Autodesk Fusion 360 part; units mm, degrees
note: some values were not read from the file. Chosen so that the rebuilt part matches the saved one: which bodies a step acts on; which face or edge a step refers to. Set by a fixed rule: which sketch regions a step uses.
(part 3 of 4)
sketch "Profile (3)" plane through (0, 0, 21) normal (0, 0, 1) x (-1, 0, 0) in component "Top Plate"
  circle A0 centre (172.0478, -239.295) radius 1.5
  circle A1 centre (168.5847, -232.6424) radius 5
  circle A2 centre (165.1216, -225.9898) radius 1.5
  circle A3 centre (67, -37.5) radius 1.5
  circle A4 centre (78.7284, -60.0301) radius 1.5
  line L0 (167.0843, -250.3342) -> (183.9375, -241.5609)
  line L1 (183.9375, -241.5609) -> (73.1179, -28.6783)
  line L2 (73.1179, -28.6783) -> (56.2647, -37.4516)
  line L3 (56.2647, -37.4516) -> (167.0843, -250.3342)
  line L4 (156, -22.3832) -> (156, 22.3832)
  arc A5 (155.0534, -25.3107) -> (156, -22.3832) centre (151, -22.3832) ccw
  line L5 (150.3466, -31.8278) -> (155.0534, -25.3107)
  arc A6 (148.1584, -33.5394) -> (150.3466, -31.8278) centre (146.2932, -28.9003) ccw
  line L6 (102.5293, -51.8851) -> (148.1584, -33.5394)
  arc A7 (102.5293, -51.8851) -> (100.1362, -53.9037) centre (104.3945, -56.5242) ccw
  line L7 (94.075, -63.7531) -> (100.1362, -53.9037)
  arc A8 (91.0078, -65.9886) -> (94.075, -63.7531) centre (89.8167, -61.1326) ccw
  line L8 (68.4899, -71.5119) -> (91.0078, -65.9886)
  arc A9 (64.7398, -70.9514) -> (68.4899, -71.5119) centre (67.2988, -66.6559) ccw
  line L9 (43.9667, -58.5759) -> (64.7398, -70.9514)
  arc A10 (43.9667, -58.5759) -> (41.8797, -57.8938) centre (41.4077, -62.8714) ccw
  line L10 (-13.2682, -52.6642) -> (41.8797, -57.8938)
  arc A11 (-13.2682, -52.6642) -> (-16.4597, -53.4461) centre (-13.7403, -57.6419) ccw
  line L11 (-40.2244, -68.8491) -> (-16.4597, -53.4461)
  arc A12 (-44.0623, -69.5267) -> (-40.2244, -68.8491) centre (-42.9439, -64.6534) ccw
  line L12 (-71.0992, -63.3215) -> (-44.0623, -69.5267)
  arc A13 (-73.5163, -61.9837) -> (-71.0992, -63.3215) centre (-69.9807, -58.4482) ccw
  line L13 (-87.8503, -47.6497) -> (-73.5163, -61.9837)
  arc A14 (-87.8503, -47.6497) -> (-90.606, -46.2464) centre (-91.3858, -51.1852) ccw
  line L14 (-143.7908, -37.8488) -> (-90.606, -46.2464)
  arc A15 (-147.2125, -35.6206) -> (-143.7908, -37.8488) centre (-143.011, -32.91) ccw
  line L15 (-155.2015, -23.2377) -> (-147.2125, -35.6206)
  arc A16 (-156, -20.5271) -> (-155.2015, -23.2377) centre (-151, -20.5271) ccw
  line L16 (-156, 20.5271) -> (-156, -20.5271)
  arc A17 (-155.2015, 23.2377) -> (-156, 20.5271) centre (-151, 20.5271) ccw
  line L17 (-147.2125, 35.6206) -> (-155.2015, 23.2377)
  arc A18 (-143.7908, 37.8488) -> (-147.2125, 35.6206) centre (-143.011, 32.91) ccw
  line L18 (-90.606, 46.2464) -> (-143.7908, 37.8488)
  arc A19 (-90.606, 46.2464) -> (-87.8503, 47.6497) centre (-91.3858, 51.1852) ccw
  circle A20 centre (-90.7, 41.475) radius 1.5
  line L19 (-73.5163, 61.9837) -> (-87.8503, 47.6497)
  arc A21 (-71.0992, 63.3215) -> (-73.5163, 61.9837) centre (-69.9807, 58.4482) ccw
  line L20 (-44.0623, 69.5267) -> (-71.0992, 63.3215)
  circle A22 centre (-56.2284, 60.0301) radius 1.5
  circle A23 centre (-44.5, 37.5) radius 1.5
  arc A24 (-40.2244, 68.8491) -> (-44.0623, 69.5267) centre (-42.9439, 64.6534) ccw
  line L21 (-16.4597, 53.4461) -> (-40.2244, 68.8491)
  arc A25 (-16.4597, 53.4461) -> (-13.2682, 52.6642) centre (-13.7403, 57.6419) ccw
  line L22 (41.8797, 57.8938) -> (-13.2682, 52.6642)
  arc A26 (41.8797, 57.8938) -> (43.9667, 58.5759) centre (41.4077, 62.8714) ccw
  line L23 (64.7398, 70.9514) -> (43.9667, 58.5759)
  arc A27 (68.4899, 71.5119) -> (64.7398, 70.9514) centre (67.2988, 66.6559) ccw
  line L24 (91.0078, 65.9886) -> (68.4899, 71.5119)
  arc A28 (94.075, 63.7531) -> (91.0078, 65.9886) centre (89.8167, 61.1326) ccw
  line L25 (100.1362, 53.9037) -> (94.075, 63.7531)
  circle A29 centre (78.7284, 60.0301) radius 1.5
  circle A30 centre (67, 37.5) radius 1.5
  arc A31 (100.1362, 53.9037) -> (102.5293, 51.8851) centre (104.3945, 56.5242) ccw
  line L26 (148.1584, 33.5394) -> (102.5293, 51.8851)
  circle A32 centre (101.7, 47.55) radius 1.5
  arc A33 (150.3466, 31.8278) -> (148.1584, 33.5394) centre (146.2932, 28.9003) ccw
  line L27 (155.0534, 25.3107) -> (150.3466, 31.8278)
  arc A34 (156, 22.3832) -> (155.0534, 25.3107) centre (151, 22.3832) ccw
  circle A35 centre (151.35, 22.65) radius 1.5
  circle A36 centre (151.35, -22.65) radius 1.5
  circle A37 centre (101.7, -47.55) radius 1.5
  circle A38 centre (78.7284, -60.0301) radius 1.5
  circle A39 centre (67, -37.5) radius 1.5
  circle A40 centre (-44.5, -37.5) radius 1.5
  circle A41 centre (-56.2284, -60.0301) radius 1.5
  circle A42 centre (-90.7, -41.475) radius 1.5
  circle A43 centre (-151.5, -21.3) radius 1.5
  circle A44 centre (-151.5, 21.3) radius 1.5
  line L28 (155.6622, 0) -> (-156.3378, 0) construction
  line L29 (52, 0) -> (52, -20.8972)
  line L30 (49.8679, -24.9929) -> (34.3684, -35.8458)
  line L31 (31.5005, -36.75) -> (-11.9635, -36.75)
  line L32 (-13.7553, -36.4179) -> (-40.2918, -26.2315)
  line L33 (-43.5, -21.5636) -> (-43.5, 0)
  arc A45 (-43.5, -21.5636) -> (-40.2918, -26.2315) centre (-38.5, -21.5636) ccw
  arc A46 (-13.7553, -36.4179) -> (-11.9635, -36.75) centre (-11.9635, -31.75) ccw
  arc A47 (31.5005, -36.75) -> (34.3684, -35.8458) centre (31.5005, -31.75) ccw
  arc A48 (49.8679, -24.9929) -> (52, -20.8972) centre (47, -20.8972) ccw
  line L34 (52, 0) -> (52, 20.8972)
  arc A49 (52, 20.8972) -> (49.8679, 24.9929) centre (47, 20.8972) ccw
  line L35 (49.8679, 24.9929) -> (34.3684, 35.8458)
  arc A50 (34.3684, 35.8458) -> (31.5005, 36.75) centre (31.5005, 31.75) ccw
  line L36 (31.5005, 36.75) -> (-11.9635, 36.75)
  arc A51 (-11.9635, 36.75) -> (-13.7553, 36.4179) centre (-11.9635, 31.75) ccw
  line L37 (-13.7553, 36.4179) -> (-40.2918, 26.2315)
  arc A52 (-40.2918, 26.2315) -> (-43.5, 21.5636) centre (-38.5, 21.5636) ccw
  line L38 (-43.5, 21.5636) -> (-43.5, 0)
  circle A53 centre (151.35, 22.65) radius 3.2
  circle A54 centre (151.35, 22.65) radius 1.7
  circle A55 centre (151.35, -22.65) radius 3.2
  circle A56 centre (151.35, -22.65) radius 1.7
  circle A57 centre (101.7, 47.55) radius 3.2
  circle A58 centre (101.7, 47.55) radius 1.7
  circle A59 centre (-90.7, 41.475) radius 3.2
  circle A60 centre (-90.7, 41.475) radius 1.7
  circle A61 centre (-151.5, 21.3) radius 3.2
  circle A62 centre (-151.5, 21.3) radius 1.7
  circle A63 centre (-151.5, -21.3) radius 3.2
  circle A64 centre (-151.5, -21.3) radius 1.7
  circle A65 centre (-90.7, -41.475) radius 3.2
  circle A66 centre (-90.7, -41.475) radius 1.7
  circle A67 centre (101.7, -47.55) radius 3.2
  circle A68 centre (101.7, -47.55) radius 1.7
  point P0 (52, -23.5)
  point P1 (-43.5, -25)
  dimension "d210" = 95.5
  dimension "d211" = 43.5
  dimension "d212" = 36.75
  dimension "d213" = 25
  dimension "d214" = 23.5
  dimension "d215" = 145
  dimension "d216" = 159
  dimension "d217" = 5
  dimension "d218" = 5
  dimension "d219" = 5
  dimension "d220" = 5
  dimension "d339" = 6.4
  dimension "d340" = 3.4
  dimension "d341" = 6.4
  dimension "d342" = 3.4
  dimension "d343" = 6.4
  dimension "d344" = 3.4
  dimension "d345" = 6.4
  dimension "d346" = 3.4
  dimension "d347" = 6.4
  dimension "d348" = 3.4
  dimension "d349" = 6.4
  dimension "d350" = 3.4
  dimension "d351" = 6.4
  dimension "d352" = 3.4
  dimension "d353" = 6.4
  dimension "d354" = 3.4
  constraint coincident origin L28
  constraint coincident L28 L29.start
  constraint coincident L28 L33.end
  constraint vertical L29
  constraint vertical L33
  constraint horizontal L31
  constraint coincident P1 L32
  constraint coincident P1 L33
  constraint tangent L32 A45
  constraint tangent L33 A45
  constraint tangent L31 A46
  constraint tangent L32 A46
  constraint tangent L30 A47
  constraint tangent L31 A47
  constraint coincident P0 L29
  constraint coincident P0 L30
  constraint tangent L29 A48
  constraint tangent L30 A48
  constraint symmetric L28 L29.start L34.start
  constraint symmetric L28 L33.end L38.end
  constraint symmetric L28 L32.end L37.end
  constraint symmetric L28 L33.start A52.end
  constraint symmetric L28 A45 A52
  constraint symmetric L28 L31.end L36.end
  constraint symmetric L28 L32.start A51.end
  constraint symmetric L28 A46 A51
  constraint symmetric L28 L30.end L35.end
  constraint symmetric L28 L31.start A50.end
  constraint symmetric L28 A47 A50
  constraint symmetric L28 L29.end L34.end
  constraint symmetric L28 L30.start A49.end
  constraint symmetric L28 A48 A49
  constraint concentric A35 A53
  constraint concentric A53 A54
  constraint concentric A36 A55
  constraint concentric A55 A56
  constraint concentric A32 A57
  constraint concentric A57 A58
  constraint concentric A20 A59
  constraint concentric A59 A60
  constraint concentric A44 A61
  constraint concentric A61 A62
  constraint concentric A43 A63
  constraint concentric A63 A64
  constraint concentric A42 A65
  constraint concentric A65 A66
  constraint concentric A37 A67
  constraint concentric A67 A68
  measures "d210" distance of P0 L33
  measures "d211" distance of origin L33
  measures "d212" distance of L28 L31
  measures "d213" distance of P1 L33.end
  measures "d214" distance of L29.start P0
  measures "d215" angle of L30 L31
  measures "d216" angle of L31 L32
  measures "d217" radius of A45
  measures "d218" radius of A46
  measures "d219" radius of A47
  measures "d220" radius of A48
  measures "d339" diameter of A53
  measures "d340" diameter of A54
  measures "d341" diameter of A55
  measures "d342" diameter of A56
  measures "d343" diameter of A57
  measures "d344" diameter of A58
  measures "d345" diameter of A59
  measures "d346" diameter of A60
  measures "d347" diameter of A61
  measures "d348" diameter of A62
  measures "d349" diameter of A63
  measures "d350" diameter of A64
  measures "d351" diameter of A65
  measures "d352" diameter of A66
  measures "d353" diameter of A67
  measures "d354" diameter of A68
extrude "Extrude1''''" add sketch "Profile (3)" along normal blind 2 separate body contours L1 L2 L3 L4 A5 L5 A6 L6 A7 L7 A8 L8 A9 L9 A10 L10 A11 L11 A12 L12 A13 L13 A14 L14 A15 L15 A16 L16 A17 L17 A18 L18 A19 L19 A21 L20 A24 L21 A25 L22 A26 L23 A27 L24 A28 L25 A31 L26 A33 L27 A34 | L1 L2 L3 A8 L8 | A53 | A54 | A55 | A56 | A57 | A58 | A59 | A60 | A61 | A62 | A63 | A64 | A65 | A66 | A67 | A68 makes body 39 in component "Top Plate"
ref_plane "WorkPlane1" through (0, 0, 33) normal (0, 0, 1) x (-1, 0, 0)
ref_plane "WorkPlane2" through (0, 0, 50) normal (0, 0, 1) x (-1, 0, 0)
sketch "Profile (4)" plane through (0, 0, 33) normal (0, 0, 1) x (1, 0, 0) in component "Pixhawk Plate"
  line L0 (-96.5, 0) -> (76.5, 0) construction
  line L1 (-96.5, 0) -> (-96.5, 20.5093)
  line L2 (-95.8379, 21.9959) -> (-82.5, 34)
  line L3 (-82.5, 34) -> (-79.0886, 42.1448)
  line L4 (-77.0182, 43.9038) -> (-62.67, 47.3296)
  line L5 (-58.958, 46.7668) -> (-50.5, 41.75)
  line L6 (-50.5, 41.75) -> (17.5, 36.3)
  line L7 (17.5, 36.3) -> (35.25, 47.75)
  line L8 (35.25, 47.75) -> (38.75, 47.75)
  line L9 (38.75, 47.75) -> (51.4852, 44.6807)
  line L10 (52.952, 43.2406) -> (55.75, 32.5)
  line L11 (55.75, 32.5) -> (76.5, 21)
  line L12 (76.5, 21) -> (76.5, 0)
  arc A0 (-95.8379, 21.9959) -> (-96.5, 20.5093) centre (-94.5, 20.5093) ccw
  arc A1 (-77.0182, 43.9038) -> (-79.0886, 42.1448) centre (-76.3215, 40.9858) ccw
  arc A2 (-58.958, 46.7668) -> (-62.67, 47.3296) centre (-61.5088, 42.4663) ccw
  arc A3 (52.952, 43.2406) -> (51.4852, 44.6807) centre (51.0166, 42.7364) ccw
  circle A4 centre (-67, 37.5) radius 1.5
  circle A5 centre (44.5, 37.5) radius 1.5
  circle A6 centre (44.5, -37.5) radius 1.5
  circle A7 centre (-67, -37.5) radius 1.5
  line L13 (-80.8, 26.9) -> (-67.05, 26.9)
  line L14 (-67.05, 22.65) -> (-80.8, 22.65)
  line L15 (-25.375, 30.5) -> (-7.875, 30.5)
  line L16 (-7.875, 26.25) -> (-25.375, 26.25)
  line L17 (4.975, 30.5) -> (17.375, 30.5)
  line L18 (17.375, 26.25) -> (4.975, 26.25)
  line L19 (43.3, 24.8) -> (59.3, 24.8)
  line L20 (59.3, 20.55) -> (43.3, 20.55)
  line L21 (32.35, 0) -> (32.35, 20.5)
  line L22 (37.1, 20.5) -> (37.1, 0)
  line L23 (-59, 0) -> (-59, 20)
  line L24 (-54.25, 20) -> (-54.25, 0)
  circle A8 centre (-42.25, 34) radius 1.5
  circle A9 centre (28.4, 34) radius 1.5
  circle A10 centre (39.175, 41.335) radius 1.5
  arc A11 (59.3, 20.55) -> (59.3, 24.8) centre (59.3, 22.675) ccw
  arc A12 (43.3, 24.8) -> (43.3, 20.55) centre (43.3, 22.675) ccw
  arc A13 (37.1, 20.5) -> (32.35, 20.5) centre (34.725, 20.5) ccw
  arc A14 (-25.375, 30.5) -> (-25.375, 26.25) centre (-25.375, 28.375) ccw
  arc A15 (-7.875, 26.25) -> (-7.875, 30.5) centre (-7.875, 28.375) ccw
  arc A16 (4.975, 30.5) -> (4.975, 26.25) centre (4.975, 28.375) ccw
  arc A17 (17.375, 26.25) -> (17.375, 30.5) centre (17.375, 28.375) ccw
  arc A18 (-80.8, 26.9) -> (-80.8, 22.65) centre (-80.8, 24.775) ccw
  arc A19 (-67.05, 22.65) -> (-67.05, 26.9) centre (-67.05, 24.775) ccw
  arc A20 (-54.25, 20) -> (-59, 20) centre (-56.625, 20) ccw
  line L25 (-42.25, 34) -> (28.4, 34) construction
  arc A21 (-59, -20) -> (-54.25, -20) centre (-56.625, -20) ccw
  line L26 (-7.875, -26.25) -> (-25.375, -26.25)
  line L27 (-54.25, -20) -> (-54.25, 0)
  line L28 (35.25, -47.75) -> (38.75, -47.75)
  line L29 (-50.5, -41.75) -> (17.5, -36.3)
  arc A22 (59.3, -24.8) -> (59.3, -20.55) centre (59.3, -22.675) ccw
  circle A23 centre (-42.25, -34) radius 1.5
  line L30 (-42.25, -34) -> (28.4, -34) construction
  arc A24 (32.35, -20.5) -> (37.1, -20.5) centre (34.725, -20.5) ccw
  arc A25 (-79.0886, -42.1448) -> (-77.0182, -43.9038) centre (-76.3215, -40.9858) ccw
  arc A26 (4.975, -26.25) -> (4.975, -30.5) centre (4.975, -28.375) ccw
  line L31 (32.35, 0) -> (32.35, -20.5)
  line L32 (-58.958, -46.7668) -> (-50.5, -41.75)
  line L33 (-77.0182, -43.9038) -> (-62.67, -47.3296)
  arc A27 (-67.05, -26.9) -> (-67.05, -22.65) centre (-67.05, -24.775) ccw
  line L34 (-59, 0) -> (-59, -20)
  arc A28 (-25.375, -26.25) -> (-25.375, -30.5) centre (-25.375, -28.375) ccw
  line L35 (-96.5, 0) -> (-96.5, -20.5093)
  arc A29 (-62.67, -47.3296) -> (-58.958, -46.7668) centre (-61.5088, -42.4663) ccw
  line L36 (-25.375, -30.5) -> (-7.875, -30.5)
  arc A30 (-80.8, -22.65) -> (-80.8, -26.9) centre (-80.8, -24.775) ccw
  arc A31 (43.3, -20.55) -> (43.3, -24.8) centre (43.3, -22.675) ccw
  circle A32 centre (44.5, -37.5) radius 1.5
  line L37 (4.975, -30.5) -> (17.375, -30.5)
  arc A33 (17.375, -30.5) -> (17.375, -26.25) centre (17.375, -28.375) ccw
  arc A34 (-7.875, -30.5) -> (-7.875, -26.25) centre (-7.875, -28.375) ccw
  circle A35 centre (28.4, -34) radius 1.5
  line L38 (59.3, -20.55) -> (43.3, -20.55)
  line L39 (37.1, -20.5) -> (37.1, 0)
  line L40 (-67.05, -22.65) -> (-80.8, -22.65)
  circle A36 centre (-67, -37.5) radius 1.5
  arc A37 (-96.5, -20.5093) -> (-95.8379, -21.9959) centre (-94.5, -20.5093) ccw
  line L41 (-80.8, -26.9) -> (-67.05, -26.9)
  line L42 (17.5, -36.3) -> (35.25, -47.75)
  line L43 (-82.5, -34) -> (-79.0886, -42.1448)
  line L44 (76.5, -21) -> (76.5, 0)
  arc A38 (51.4852, -44.6807) -> (52.952, -43.2406) centre (51.0166, -42.7364) ccw
  line L45 (55.75, -32.5) -> (76.5, -21)
  line L46 (52.952, -43.2406) -> (55.75, -32.5)
  line L47 (43.3, -24.8) -> (59.3, -24.8)
  circle A39 centre (39.175, -41.335) radius 1.5
  line L48 (38.75, -47.75) -> (51.4852, -44.6807)
  line L49 (-95.8379, -21.9959) -> (-82.5, -34)
  line L50 (17.375, -26.25) -> (4.975, -26.25)
  circle A40 centre (-67, 37.5) radius 2.75 construction
  line L51 (-67, 40.25) -> (-67, 34.75) construction
  line L52 (-64.25, 37.5) -> (-69.75, 37.5) construction
  line L53 (-64.6184, 38.875) -> (-64.6184, 36.125)
  line L54 (-67, 34.75) -> (-64.6184, 36.125)
  line L55 (-64.6184, 38.875) -> (-67, 40.25)
  line L56 (-69.3816, 38.875) -> (-69.3816, 36.125)
  line L57 (-69.3816, 38.875) -> (-67, 40.25)
  line L58 (-67, 34.75) -> (-69.3816, 36.125)
  circle A41 centre (-67, 37.5) radius 1.25
  line L59 (46.8816, 38.875) -> (44.5, 40.25)
  line L60 (42.1184, 38.875) -> (44.5, 40.25)
  line L61 (44.5, 34.75) -> (42.1184, 36.125)
  line L62 (44.5, 40.25) -> (44.5, 34.75) construction
  line L63 (46.8816, 38.875) -> (46.8816, 36.125)
  circle A42 centre (44.5, 37.5) radius 2.75 construction
  circle A43 centre (44.5, 37.5) radius 1.25
  line L64 (47.25, 37.5) -> (41.75, 37.5) construction
  line L65 (42.1184, 38.875) -> (42.1184, 36.125)
  line L66 (44.5, 34.75) -> (46.8816, 36.125)
  line L67 (-67, -34.75) -> (-67, -40.25) construction
  line L68 (-69.3816, -36.125) -> (-67, -34.75)
  line L69 (-64.25, -37.5) -> (-69.75, -37.5) construction
  circle A44 centre (-67, -37.5) radius 2.75 construction
  line L70 (-69.3816, -36.125) -> (-69.3816, -38.875)
  line L71 (-64.6184, -36.125) -> (-67, -34.75)
  line L72 (-67, -40.25) -> (-64.6184, -38.875)
  line L73 (-67, -40.25) -> (-69.3816, -38.875)
  circle A45 centre (-67, -37.5) radius 1.25
  line L74 (-64.6184, -36.125) -> (-64.6184, -38.875)
  line L75 (44.5, -34.75) -> (44.5, -40.25) construction
  line L76 (42.1184, -36.125) -> (44.5, -34.75)
  line L77 (46.8816, -36.125) -> (44.5, -34.75)
  line L78 (46.8816, -36.125) -> (46.8816, -38.875)
  line L79 (44.5, -40.25) -> (46.8816, -38.875)
  line L80 (44.5, -40.25) -> (42.1184, -38.875)
  circle A46 centre (44.5, -37.5) radius 1.25
  line L81 (47.25, -37.5) -> (41.75, -37.5) construction
  line L82 (42.1184, -36.125) -> (42.1184, -38.875)
  circle A47 centre (44.5, -37.5) radius 1.5
  circle A48 centre (44.5, -37.5) radius 2.75 construction
  point P0 (-96.5, 21.4)
  point P1 (-78.5, 43.55)
  point P2 (-60.7, 47.8)
  point P3 (52.65, 44.4)
  point P4 (-60.7, -47.8)
  point P5 (-78.5, -43.55)
  point P6 (-96.5, -21.4)
  point P7 (52.65, -44.4)
  dimension "d225" = 173
  dimension "d226" = 76.5
  dimension "d227" = 21
  dimension "d228" = 21.4
  dimension "d229" = 34
  dimension "d230" = 32.5
  dimension "d232" = 47.75
  dimension "d233" = 37.75
  dimension "d234" = 41.25
  dimension "d235" = 20.75
  dimension "d236" = 44.4
  dimension "d237" = 23.85
  dimension "d238" = 17.5
  dimension "d239" = 50.5
  dimension "d240" = 14
  dimension "d241" = 43.55
  dimension "d242" = 47.8
  dimension "d243" = 18
  dimension "d244" = 35.8
  dimension "d245" = 41.75
  dimension "d246" = 36.3
  dimension "d247" = 2
  dimension "d248" = 3
  dimension "d249" = 5
  dimension "d250" = 2
  dimension "d251" = 3
  dimension "d252" = 3
  dimension "d253" = 3
  dimension "d254" = 4.25
  dimension "d255" = 13.75
  dimension "d256" = 4.75
  dimension "d257" = 4.25
  dimension "d258" = 17.5
  dimension "d259" = 12.4
  dimension "d260" = 4.25
  dimension "d261" = 4.75
  dimension "d262" = 20.5
  dimension "d263" = 20
  dimension "d264" = 54.25
  dimension "d265" = 32.35
  dimension "d266" = 26.25
  dimension "d267" = 12.85
  dimension "d268" = 22.65
  dimension "d269" = 34
  dimension "d270" = 70.65
  dimension "d271" = 28.4
  dimension "d272" = 16
  dimension "d273" = 20.55
  dimension "d274" = 17.2
  dimension "d275" = 3.835
  dimension "d276" = 5.325
  dimension "d277" = 17.375
  dimension "d278" = 15.7
  dimension "d359" = 5.5
  dimension "d360" = 2.5
  dimension "d361" = 5.5
  dimension "d362" = 2.5
  dimension "d363" = 5.5
  dimension "d364" = 2.5
  dimension "d365" = 5.5
  dimension "d366" = 2.5
  constraint horizontal L0
  constraint coincident origin L0
  constraint vertical L1
  constraint vertical L12
  constraint horizontal L8
  constraint coincident P0 L1
  constraint coincident P0 L2
  constraint tangent L1 A0
  constraint tangent L2 A0
  constraint coincident P1 L3
  constraint coincident P1 L4
  constraint tangent L3 A1
  constraint tangent L4 A1
  constraint coincident P2 L4
  constraint coincident P2 L5
  constraint tangent L4 A2
  constraint tangent L5 A2
  constraint coincident P3 L9
  constraint coincident P3 L10
  constraint tangent L9 A3
  constraint tangent L10 A3
  constraint horizontal L13
  constraint horizontal L14
  constraint horizontal L15
  constraint horizontal L16
  constraint horizontal L17
  constraint horizontal L18
  constraint horizontal L19
  constraint horizontal L20
  constraint coincident L0 L21.start
  constraint coincident L0 L22.end
  constraint vertical L22
  constraint vertical L21
  constraint coincident L0 L23.start
  constraint coincident L0 L24.end
  constraint vertical L23
  constraint vertical L24
  constraint tangent L14 A18
  constraint tangent L14 A19
  constraint tangent L24 A20
  constraint tangent L16 A14
  constraint tangent L16 A15
  constraint tangent L18 A16
  constraint tangent L18 A17
  constraint tangent L22 A13
  constraint tangent L20 A12
  constraint tangent L20 A11
  constraint tangent L19 A11
  constraint tangent L19 A12
  constraint tangent L21 A13
  constraint tangent L15 A14
  constraint tangent L17 A16
  constraint tangent L13 A18
  constraint tangent L13 A19
  constraint tangent L23 A20
  constraint collinear L15 L17
  constraint collinear L16 L18
  constraint tangent L15 A15
  constraint coincident A8.centre L25.start
  constraint coincident A9.centre L25.end
  constraint horizontal L25
  constraint tangent L17 A17
  constraint symmetric L1.start L0 L35.start
  constraint symmetric L12.end L0 L44.end
  constraint symmetric L0 P0 P6
  constraint symmetric L0 L2.end L43.start
  constraint symmetric L0 P1 P5
  constraint symmetric L0 P2 P4
  constraint symmetric L0 L5.end L29.start
  constraint symmetric L0 L6.end L29.end
  constraint symmetric L0 L7.end L28.start
  constraint symmetric L0 L8.end L28.end
  constraint symmetric L0 P3 P7
  constraint symmetric L0 L10.end L45.start
  constraint symmetric L0 L11.end L44.start
  constraint symmetric L0 L1.end L35.end
  constraint symmetric L0 L2.start A37.end
  constraint symmetric L0 A0 A37
  constraint symmetric L0 L3.end A25.start
  constraint symmetric L0 L4.start A25.end
  constraint symmetric L0 A1 A25
  constraint symmetric L0 L4.end L33.end
  constraint symmetric L0 L5.start L32.start
  constraint symmetric L0 A2 A29
  constraint symmetric L0 L9.end A38.start
  constraint symmetric L0 L10.start A38.end
  constraint symmetric L0 A3 A38
  constraint symmetric L0 A4 A36
  constraint symmetric L0 A5 A32
  constraint symmetric L0 L13.start A30.end
  constraint symmetric L0 L13.end A27.start
  constraint symmetric L0 L14.start A27.end
  constraint symmetric L0 L14.end A30.start
  constraint symmetric L0 L15.start A28.end
  constraint symmetric L0 L15.end L36.end
  constraint symmetric L0 L16.start L26.start
  constraint symmetric L0 L16.end L26.end
  constraint symmetric L0 L17.start A26.end
  constraint symmetric L0 L17.end L37.end
  constraint symmetric L0 L18.start A33.end
  constraint symmetric L0 L18.end A26.start
  constraint symmetric L0 L19.start A31.end
  constraint symmetric L0 L19.end A22.start
  constraint symmetric L0 L20.start A22.end
  constraint symmetric L0 L20.end A31.start
  constraint symmetric L0 L21.start L31.start
  constraint symmetric L0 L21.end A24.start
  constraint symmetric L0 L22.start A24.end
  constraint symmetric L0 L22.end L39.end
  constraint symmetric L0 L23.start L34.start
  constraint symmetric L0 L23.end A21.start
  constraint symmetric L0 L24.start A21.end
  constraint symmetric L0 L24.end L27.end
  constraint symmetric L0 A8 A23
  constraint symmetric L0 A9 A35
  constraint symmetric L0 A10 A39
  constraint symmetric L0 A11 A22
  constraint symmetric L0 A12 A31
  constraint symmetric L0 A13 A24
  constraint symmetric L0 A14 A28
  constraint symmetric L0 A15 A34
  constraint symmetric L0 A16 A26
  constraint symmetric L0 A17 A33
  constraint symmetric L0 A18 A30
  constraint symmetric L0 A19 A27
  constraint symmetric L0 A20 A21
  constraint symmetric L0 A8.centre A23.centre
  constraint symmetric L0 A9.centre L30.end
  constraint concentric A4 A40
  constraint coincident A40 L51.start
  constraint coincident A40 L51.end
  constraint vertical L51
  constraint coincident A40 L52.start
  constraint coincident A40 L52.end
  constraint perpendicular L51 L52
  constraint coincident A4.centre L51
  constraint coincident A4.centre L52
  constraint coincident A40 L53.start
  constraint coincident A40 L53.end
  constraint vertical L53
  constraint coincident A40 L56.start
  constraint coincident A40 L56.end
  constraint vertical L56
  constraint equal L53 L55
  constraint equal L55 L57
  constraint concentric A40 A41
  constraint coincident L59.end A42
  constraint coincident L61.start A42
  constraint vertical L62
  constraint coincident L64.start A42
  constraint coincident L64.end A42
  constraint perpendicular L62 L64
  constraint coincident A5.centre L62
  constraint coincident A5.centre L64
  constraint coincident L59.start A42
  constraint coincident L63.end A42
  constraint vertical L63
  constraint coincident L60.start A42
  constraint coincident L61.end A42
  constraint vertical L65
  constraint equal L59 L63
  constraint equal L59 L60
  constraint concentric A42 A43
  constraint coincident A5.centre A42.centre
  constraint coincident L67.start A44
  constraint coincident L67.end A44
  constraint vertical L67
  constraint coincident L69.start A44
  constraint coincident L69.end A44
  constraint perpendicular L67 L69
  constraint coincident A7.centre L67
  constraint coincident A7.centre L69
  constraint coincident L71.start A44
  constraint coincident L72.end A44
  constraint vertical L74
  constraint coincident L68.start A44
  constraint coincident L70.end A44
  constraint vertical L70
  constraint equal L71 L74
  constraint equal L68 L71
  constraint concentric A44 A45
  constraint coincident A7.centre A36.centre
  constraint coincident L75.start A48
  constraint coincident L75.end A48
  constraint vertical L75
  constraint coincident L81.start A48
  constraint coincident L81.end A48
  constraint perpendicular L75 L81
  constraint coincident A6.centre L75
  constraint coincident A6.centre L81
  constraint coincident L77.start A48
  constraint coincident L78.end A48
  constraint vertical L78
  constraint coincident L76.start A48
  constraint coincident L80.end A48
  constraint vertical L82
  constraint equal L77 L78
  constraint equal L76 L77
  constraint concentric A46 A48
  constraint coincident A6.centre A32.centre
  measures "d225" distance of L1 L12
  measures "d226" distance of origin L12
  measures "d227" distance of L0.end L11.end
  measures "d228" distance of L0.start P0
  measures "d229" distance of L0 L2.end
  measures "d230" distance of L0 L10.end
  measures "d232" distance of L0 L8
  measures "d233" distance of L8.end L12
  measures "d234" distance of L7.end L12
  measures "d235" distance of L10.end L12
  measures "d236" distance of L0 P3
  measures "d237" distance of P3 L12
  measures "d238" horizontal distance of origin L6.end
  measures "d239" horizontal distance of origin L5.end
  measures "d240" distance of L1 L2.end
  measures "d241" distance of L0 P1
  measures "d242" distance of L0 P2
  measures "d243" distance of L1 P1
  measures "d244" distance of L1 P2
  measures "d245" vertical distance of origin L5.end
  measures "d246" vertical distance of origin L6.end
  measures "d247" radius of A0
  measures "d248" radius of A1
  measures "d249" radius of A2
  measures "d250" radius of A3
  measures "d251" diameter of A8
  measures "d252" diameter of A9
  measures "d253" diameter of A10
  measures "d254" distance of L13 L14
  measures "d255" distance of A18.centre A19.centre
  measures "d256" distance of L23 L24
  measures "d257" distance of L15 L16
  measures "d258" horizontal distance of A14.centre A15.centre
  measures "d259" distance of A16.centre A17.centre
  measures "d260" distance of L19 L20
  measures "d261" distance of L21 L22
  measures "d262" distance of L0 A13.centre
  measures "d263" distance of L0 A20.centre
  measures "d264" distance of origin L24
  measures "d265" distance of origin L21
  measures "d266" distance of L0 L16
  measures "d267" distance of A15.centre A16.centre
  measures "d268" distance of L0 L14
  measures "d269" distance of L0 A8.centre
  measures "d270" distance of A8.centre A9.centre
  measures "d271" horizontal distance of origin A9.centre
  measures "d272" distance of A12.centre A11.centre
  measures "d273" distance of L0 L20
  measures "d274" distance of L12 A11.centre
  measures "d275" vertical distance of A5.centre A10.centre
  measures "d276" horizontal distance of A5.centre A10.centre
  measures "d277" horizontal distance of origin A17.centre
  measures "d278" distance of L1 A18.centre
  measures "d359" diameter of A40
  measures "d360" diameter of A41
  measures "d361" diameter of A42
  measures "d362" diameter of A43
  measures "d363" diameter of A44
  measures "d364" diameter of A45
  measures "d365" diameter of A48
  measures "d366" diameter of A46
extrude "Extrude1'''''" add sketch "Profile (4)" along normal blind 2 separate body contours L1 L2 L3 L4 L5 L6 L7 L8 L9 L10 L11 L12 A0 A1 A2 A3 L28 L29 A25 L32 L33 L35 A29 A37 L42 L43 L44 A38 L45 L46 L48 L49 | L53 L54 L55 L56 L57 L58 | L59 L60 L61 L63 L65 L66 | L68 L70 L71 L72 L73 L74 | L76 L77 L78 L79 L80 L82 makes body 40 in component "Pixhawk Plate"
sketch "Profile (5)" plane through (0, 0, 50) normal (0, 0, 1) x (1, 0, 0) in component "Accessory Plate"
  circle A0 centre (-42.25, 34) radius 1.5
  circle A1 centre (-42.25, -34) radius 1.5
  circle A2 centre (28.4, -34) radius 1.5
  circle A3 centre (28.4, 34) radius 1.5
  line L0 (-70.5, 0) -> (75, 0) construction
  line L1 (-70.5, 0) -> (-70.5, 12.5)
  line L2 (-70.5, 12.5) -> (-54.7221, 33.4587)
  line L3 (-52.2059, 35.2279) -> (-43.25, 38)
  line L4 (-43.25, 38) -> (-31.65, 38)
  line L5 (-31.65, 38) -> (-27.15, 33.5)
  line L6 (-27.15, 33.5) -> (9.25, 33.5)
  line L7 (9.25, 33.5) -> (13.75, 38)
  line L8 (13.75, 38) -> (30, 38)
  line L9 (30, 38) -> (42, 26.25)
  line L10 (42, 26.25) -> (70.822, 21.4463)
  line L11 (75, 16.5144) -> (75, 0)
  arc A4 (-52.2059, 35.2279) -> (-54.7221, 33.4587) centre (-50.7275, 30.4515) ccw
  arc A5 (75, 16.5144) -> (70.822, 21.4463) centre (70, 16.5144) ccw
  circle A6 centre (-50.25, 29.25) radius 4
  line L12 (-56.2, 0) -> (-56.2, 11.1318)
  line L13 (-55.4036, 12.729) -> (-46.75, 19.25)
  line L14 (-46.75, 19.25) -> (-36.9216, 19.25)
  line L15 (-47.8662, 1.6509) -> (-34.9726, 14.5445)
  line L16 (-32.5282, 1.6218) -> (-14.9, 19.25)
  line L17 (-5.6636, 14.8105) -> (-18.5125, 1.9617)
  line L18 (-3.4193, 1.5227) -> (13.4941, 18.4361)
  line L19 (19.5897, 14.4044) -> (19.5897, 0)
  line L20 (-24.8, 24.75) -> (8, 24.75)
  line L21 (-26.2737, 29) -> (9.4737, 29)
  circle A7 centre (37.85, 16) radius 1.5
  circle A8 centre (69.85, 16) radius 1.5
  line L22 (37.85, 16) -> (69.85, 16) construction
  line L23 (-24.8, 24.75) -> (-27.0868, 27.0368)
  line L24 (8, 24.75) -> (10.2868, 27.0368)
  arc A9 (10.2868, 27.0368) -> (9.4737, 29) centre (9.4737, 27.85) ccw
  arc A10 (-26.2737, 29) -> (-27.0868, 27.0368) centre (-26.2737, 27.85) ccw
  line L25 (-48.55, 0) -> (-48.55, 5.3896) construction
  arc A11 (-47.8662, 1.6509) -> (-48.55, 0) centre (-46.2153, 0) ccw
  arc A12 (-34.9726, 14.5445) -> (-36.9216, 19.25) centre (-36.9216, 16.4936) ccw
  arc A13 (-55.4036, 12.729) -> (-56.2, 11.1318) centre (-54.2, 11.1318) ccw
  arc A14 (-32.5282, 1.6218) -> (-33.2, 0) centre (-30.9065, 0) ccw
  line L26 (-33.2, 0) -> (-33.2, 5.3774) construction
  line L27 (-19.325, 0) -> (-19.325, 2.9872) construction
  arc A15 (-18.5125, 1.9617) -> (-19.325, 0) centre (-16.5508, 0) ccw
  line L28 (-4.05, 0) -> (-4.05, 2.1317) construction
  arc A16 (-3.4193, 1.5227) -> (-4.05, 0) centre (-1.8966, 0) ccw
  line L29 (-14.9, 19.25) -> (-7.5026, 19.25)
  arc A17 (-5.6636, 14.8105) -> (-7.5026, 19.25) centre (-7.5026, 16.6494) ccw
  spline S0 degree 5 poles (13.4941, 18.4361) (13.5655, 18.5075) (13.7132, 18.651) (13.9496, 18.869) (14.3035, 19.15) (14.8512, 19.4045) (15.5396, 19.4698) (16.3722, 19.2715) (17.2898, 18.7896) (18.1939, 18.0372) (18.9671, 17.0431) (19.3888, 16.0795) (19.5532, 15.2733) (19.5897, 14.7) (19.5897, 14.4044) knots 0 0 0 0 0 0 0.1 0.2 0.3 0.4 0.5 0.6 0.7 0.8 0.9 1 1 1 1 1 1
  line L30 (19.5897, 15.6342) -> (19.5897, 13.1745)
  line L31 (12.8985, 17.8405) -> (14.0898, 19.0317)
  line L32 (-26.2737, -29) -> (9.4737, -29)
  line L33 (-24.8, -24.75) -> (8, -24.75)
  line L34 (-27.15, -33.5) -> (9.25, -33.5)
  line L35 (-4.05, 0) -> (-4.05, -2.1317) construction
  line L36 (-56.2, 0) -> (-56.2, -11.1318)
  line L37 (-24.8, -24.75) -> (-27.0868, -27.0368)
  line L38 (-19.325, 0) -> (-19.325, -2.9872) construction
  line L39 (-70.5, 0) -> (-70.5, -12.5)
  circle A18 centre (-42.25, -34) radius 1.5
  line L40 (-33.2, 0) -> (-33.2, -5.3774) construction
  line L41 (-5.6636, -14.8105) -> (-18.5125, -1.9617)
  arc A19 (-27.0868, -27.0368) -> (-26.2737, -29) centre (-26.2737, -27.85) ccw
  line L42 (-70.5, -12.5) -> (-54.7221, -33.4587)
  arc A20 (-54.7221, -33.4587) -> (-52.2059, -35.2279) centre (-50.7275, -30.4515) ccw
  arc A21 (-4.05, 0) -> (-3.4193, -1.5227) centre (-1.8966, 0) ccw
  line L43 (-47.8662, -1.6509) -> (-34.9726, -14.5445)
  line L44 (-14.9, -19.25) -> (-7.5026, -19.25)
  line L45 (12.8985, -17.8405) -> (14.0898, -19.0317)
  line L46 (13.75, -38) -> (30, -38)
  line L47 (37.85, -16) -> (69.85, -16) construction
  line L48 (-3.4193, -1.5227) -> (13.4941, -18.4361)
  line L49 (19.5897, -14.4044) -> (19.5897, 0)
  line L50 (42, -26.25) -> (70.822, -21.4463)
  arc A22 (9.4737, -29) -> (10.2868, -27.0368) centre (9.4737, -27.85) ccw
  line L51 (-32.5282, -1.6218) -> (-14.9, -19.25)
  line L52 (8, -24.75) -> (10.2868, -27.0368)
  arc A23 (-7.5026, -19.25) -> (-5.6636, -14.8105) centre (-7.5026, -16.6494) ccw
  line L53 (-46.75, -19.25) -> (-36.9216, -19.25)
  line L54 (-43.25, -38) -> (-31.65, -38)
  line L55 (-55.4036, -12.729) -> (-46.75, -19.25)
  line L56 (19.5897, -15.6342) -> (19.5897, -13.1745)
  line L57 (9.25, -33.5) -> (13.75, -38)
  arc A24 (-56.2, -11.1318) -> (-55.4036, -12.729) centre (-54.2, -11.1318) ccw
  arc A25 (-48.55, 0) -> (-47.8662, -1.6509) centre (-46.2153, 0) ccw
  line L58 (-52.2059, -35.2279) -> (-43.25, -38)
  arc A26 (-19.325, 0) -> (-18.5125, -1.9617) centre (-16.5508, 0) ccw
  arc A27 (-36.9216, -19.25) -> (-34.9726, -14.5445) centre (-36.9216, -16.4936) ccw
  line L59 (-48.55, 0) -> (-48.55, -5.3896) construction
  circle A28 centre (37.85, -16) radius 1.5
  arc A29 (70.822, -21.4463) -> (75, -16.5144) centre (70, -16.5144) ccw
  line L60 (75, -16.5144) -> (75, 0)
  spline S1 degree 5 poles (13.4941, -18.4361) (13.5655, -18.5075) (13.7132, -18.651) (13.9496, -18.869) (14.3035, -19.15) (14.8512, -19.4045) (15.5396, -19.4698) (16.3722, -19.2715) (17.2898, -18.7896) (18.1939, -18.0372) (18.9671, -17.0431) (19.3888, -16.0795) (19.5532, -15.2733) (19.5897, -14.7) (19.5897, -14.4044) knots 0 0 0 0 0 0 0.1 0.2 0.3 0.4 0.5 0.6 0.7 0.8 0.9 1 1 1 1 1 1
  line L61 (12.8985, -17.8405) -> (14.0898, -19.0317)
  line L62 (19.5897, -15.6342) -> (19.5897, -13.1745)
  line L63 (30, -38) -> (42, -26.25)
  line L64 (-31.65, -38) -> (-27.15, -33.5)
  arc A30 (-33.2, 0) -> (-32.5282, -1.6218) centre (-30.9065, 0) ccw
  circle A31 centre (28.4, -34) radius 1.5
  circle A32 centre (69.85, -16) radius 1.5
  circle A33 centre (-42.25, 34) radius 2.75 construction
  line L65 (-42.25, 36.75) -> (-42.25, 31.25) construction
  line L66 (-44.6316, 35.375) -> (-44.6316, 32.625)
  line L67 (-44.6316, 35.375) -> (-42.25, 36.75)
  circle A34 centre (-42.25, 34) radius 1.25
  line L68 (-42.25, -36.75) -> (-44.6316, -35.375)
  line L69 (-39.8684, -32.625) -> (-39.8684, -35.375)
  line L70 (-44.6316, -32.625) -> (-44.6316, -35.375)
  circle A35 centre (-42.25, -34) radius 2.75 construction
  line L71 (-44.6316, -32.625) -> (-42.25, -31.25)
  line L72 (-42.25, -36.75) -> (-39.8684, -35.375)
  circle A36 centre (-42.25, -34) radius 1.5
  line L73 (-39.8684, -32.625) -> (-42.25, -31.25)
  line L74 (-45, -34) -> (-39.5, -34) construction
  line L75 (-42.25, -31.25) -> (-42.25, -36.75) construction
  circle A37 centre (-42.25, -34) radius 1.25
  line L76 (-42.25, 31.25) -> (-39.8684, 32.625)
  line L77 (-39.8684, 35.375) -> (-39.8684, 32.625)
  line L78 (-42.25, 31.25) -> (-44.6316, 32.625)
  line L79 (-45, 34) -> (-39.5, 34) construction
  line L80 (28.4, 31.25) -> (30.7816, 32.625)
  line L81 (26.0184, 35.375) -> (28.4, 36.75)
  circle A38 centre (28.4, 34) radius 2.75 construction
  line L82 (30.7816, 35.375) -> (30.7816, 32.625)
  circle A39 centre (28.4, 34) radius 1.25
  line L83 (28.4, 31.25) -> (26.0184, 32.625)
  line L84 (25.65, 34) -> (31.15, 34) construction
  line L85 (26.0184, 35.375) -> (26.0184, 32.625)
  line L86 (30.7816, 35.375) -> (28.4, 36.75)
  line L87 (28.4, 36.75) -> (28.4, 31.25) construction
  line L88 (-42.25, 36.75) -> (-39.8684, 35.375)
  line L89 (26.0184, -32.625) -> (26.0184, -35.375)
  line L90 (28.4, -36.75) -> (26.0184, -35.375)
  line L91 (26.0184, -32.625) -> (28.4, -31.25)
  line L92 (28.4, -31.25) -> (28.4, -36.75) construction
  line L93 (30.7816, -32.625) -> (30.7816, -35.375)
  line L94 (25, -26) -> (30.5, -26) construction
  line L95 (28.4, -31.25) -> (30.7816, -32.625)
  circle A40 centre (28.4, -34) radius 1.25
  line L96 (28.4, -36.75) -> (30.7816, -35.375)
  circle A41 centre (28.4, -34) radius 2.75 construction
  point P0 (-53.75, 34.75)
  point P1 (75, 20.75)
  point P2 (15.5976, 19.4021)
  point P3 (-53.75, -34.75)
  point P4 (15.5976, -19.4021)
  point P5 (75, -20.75)
  dimension "d281" = 145.5
  dimension "d282" = 75
  dimension "d283" = 20.75
  dimension "d284" = 26.25
  dimension "d285" = 38
  dimension "d286" = 12.5
  dimension "d287" = 34.75
  dimension "d288" = 33.5
  dimension "d289" = 33
  dimension "d290" = 45
  dimension "d291" = 16.75
  dimension "d292" = 27.25
  dimension "d293" = 135
  dimension "d294" = 135
  dimension "d295" = 13.75
  dimension "d296" = 31.65
  dimension "d297" = 5
  dimension "d298" = 5
  dimension "d299" = 8
  dimension "d300" = 3
  dimension "d301" = 3
  dimension "d302" = 16
  dimension "d303" = 32
  dimension "d304" = 5.15
  dimension "d306" = 4.25
  dimension "d307" = 1.15
  dimension "d308" = 1.15
  dimension "d309" = 24.75
  dimension "d310" = 32.8
  dimension "d311" = 8
  dimension "d312" = 2
  dimension "d313" = 14.3
  dimension "d314" = 7.65
  dimension "d315" = 19.25
  dimension "d316" = 45
  dimension "d317" = 127
  dimension "d318" = 14.9
  dimension "d319" = 46.75
  dimension "d320" = 19.325
  dimension "d321" = 33.2
  dimension "d322" = 4.05
  dimension "d323" = 20.25
  dimension "d324" = 29.25
  dimension "d369" = 5.5
  dimension "d370" = 2.5
  dimension "d371" = 5.5
  dimension "d374" = 2.5
  dimension "d376" = 5.5
  dimension "d377" = 2.5
  dimension "d379" = 5.5
  dimension "d380" = 2.5
  constraint horizontal L0
  constraint coincident origin L0
  constraint vertical L11
  constraint vertical L1
  constraint horizontal L8
  constraint horizontal L4
  constraint horizontal L6
  constraint collinear L4 L8
  constraint coincident P0 L2
  constraint coincident P0 L3
  constraint tangent L2 A4
  constraint tangent L3 A4
  constraint coincident P1 L10
  constraint coincident P1 L11
  constraint tangent L10 A5
  constraint tangent L11 A5
  constraint coincident L0 L12.start
  constraint coincident L0 L19.end
  constraint horizontal L20
  constraint parallel L20 L21
  constraint coincident A7.centre L22.start
  constraint coincident A8.centre L22.end
  constraint horizontal L22
  constraint parallel L7 L24
  constraint parallel L5 L23
  constraint tangent L21 A9
  constraint tangent L24 A9
  constraint tangent L23 A10
  constraint tangent L21 A10
  constraint horizontal L14
  constraint vertical L12
  constraint coincident L0 L25.start
  constraint tangent L15 A11
  constraint vertical L25
  constraint tangent L25 A11
  constraint tangent L14 A12
  constraint tangent L15 A12
  constraint tangent L12 A13
  constraint tangent L13 A13
  constraint vertical L26
  constraint tangent A14 L26
  constraint coincident L0 A14.end
  constraint tangent L16 A14
  constraint coincident L0 L27.start
  constraint vertical L27
  constraint tangent L17 A15
  constraint tangent L27 A15
  constraint coincident L0 L28.start
  constraint vertical L28
  constraint tangent L18 A16
  constraint tangent L28 A16
  constraint horizontal L29
  constraint collinear L14 L29
  constraint parallel L15 L16
  constraint parallel L16 L17
  constraint parallel L17 L18
  constraint vertical L19
  constraint tangent L29 A17
  constraint tangent L17 A17
  constraint midpoint L19.start L30
  constraint collinear L19 L30
  constraint midpoint L18.end L31
  constraint collinear L18 L31
  constraint symmetric A0 L0 A18
  constraint symmetric A3 L0 A31
  constraint symmetric L1.start L0 L39.start
  constraint symmetric L11.end L0 L60.end
  constraint symmetric L0 L1.end L39.end
  constraint symmetric L0 P0 P3
  constraint symmetric L0 L3.end L54.start
  constraint symmetric L0 L4.end L54.end
  constraint symmetric L0 L5.end L34.start
  constraint symmetric L0 L6.end L34.end
  constraint symmetric L0 L7.end L46.start
  constraint symmetric L0 L8.end L46.end
  constraint symmetric L0 L9.end L50.start
  constraint symmetric L0 P1 P5
  constraint symmetric L0 L2.end L42.end
  constraint symmetric L0 L3.start A20.end
  constraint symmetric L0 A4 A20
  constraint symmetric L0 L10.end L50.end
  constraint symmetric L0 L11.start A29.end
  constraint symmetric L0 A5 A29
  constraint symmetric L0 L12.start L36.start
  constraint symmetric L0 L13.end L53.start
  constraint symmetric L0 L14.end L53.end
  constraint symmetric L0 L15.start L43.start
  constraint symmetric L0 L15.end L43.end
  constraint symmetric L0 L16.end L44.start
  constraint symmetric L0 L17.start L41.start
  constraint symmetric L0 L17.end L41.end
  constraint symmetric L0 L18.start A21.end
  constraint symmetric L0 L18.end L48.end
  constraint symmetric L0 L19.start L49.start
  constraint symmetric L0 L19.end L49.end
  constraint symmetric L0 L20.start L33.start
  constraint symmetric L0 L20.end L33.end
  constraint symmetric L0 A7 A28
  constraint symmetric L0 A8 A32
  constraint symmetric L0 A7.centre L47.start
  constraint symmetric L0 A8.centre L47.end
  constraint symmetric L0 L21.end L32.end
  constraint symmetric L0 L24.end A22.end
  constraint symmetric L0 A9 A22
  constraint symmetric L0 L23.end L37.end
  constraint symmetric L0 L21.start L32.start
  constraint symmetric L0 A10 A19
  constraint symmetric L0 L25.start A11.end
  constraint symmetric L0 L25.end L59.end
  constraint symmetric L0 A11 A25
  constraint symmetric L0 A12 A27
  constraint symmetric L0 L12.end L36.end
  constraint symmetric L0 L13.start L55.start
  constraint symmetric L0 A13 A24
  constraint symmetric L0 L16.start L51.start
  constraint symmetric L0 A14.end L26.start
  constraint symmetric L0 L26.end L40.end
  constraint symmetric L0 A14 A30
  constraint symmetric L0 L27.start A15.end
  constraint symmetric L0 L27.end L38.end
  constraint symmetric L0 A15 A26
  constraint symmetric L0 L28.start A16.end
  constraint symmetric L0 L28.end L35.end
  constraint symmetric L0 A16 A21
  constraint symmetric L0 L29.end L44.end
  constraint symmetric L0 A17 A23
  constraint symmetric L0 P2 P4
  constraint symmetric L0 L30.start L56.start
  constraint symmetric L0 L30.end L56.end
  constraint symmetric L0 L31.start L45.start
  constraint symmetric L0 L31.end L45.end
  constraint concentric A0 A33
  constraint coincident A33 L65.start
  constraint coincident A33 L65.end
  constraint coincident A33 L66.start
  constraint vertical L66
  constraint concentric A33 A34
  constraint coincident A35 L71.end
  constraint coincident A35 L68.start
  constraint coincident L69.start A35
  constraint coincident L69.end A35
  constraint coincident L70.start A35
  constraint coincident L68.end A35
  constraint vertical L70
  constraint vertical L69
  constraint horizontal L74
  constraint perpendicular L74 L75
  constraint horizontal L79
  constraint vertical L77
  constraint coincident L84.start A38
  constraint coincident L84.end A38
  constraint horizontal L84
  constraint coincident L81.end A38
  constraint perpendicular L84 L87
  constraint coincident L80.start A38
  constraint coincident L82.start A38
  constraint coincident L80.end A38
  constraint coincident L81.start A38
  constraint coincident L83.end A38
  constraint vertical L85
  constraint vertical L82
  constraint equal L82 L86
  constraint equal L81 L86
  constraint concentric A38 A39
  constraint coincident A3.centre A38.centre
  constraint coincident L65 A0.centre
  constraint equal L67 L88
  constraint coincident A33 L77.start
  constraint equal L77 L88
  constraint vertical L65
  constraint coincident A33 L76.end
  constraint coincident A33 L66.end
  constraint coincident L65.end L76.start
  constraint coincident L91.end A41
  constraint coincident L90.start A41
  constraint coincident L89.start A41
  constraint vertical L89
  constraint concentric A40 A41
  constraint horizontal L94
  constraint vertical L93
  constraint coincident A2.centre L92
  constraint equal L91 L95
  constraint coincident L93.start A41
  constraint equal L93 L95
  constraint vertical L92
  constraint coincident L93.end A41
  constraint coincident L89.end A41
  constraint coincident L90.start L92.end
  constraint coincident A2.centre A31.centre
  constraint coincident A1.centre L75
  constraint coincident A1.centre A18.centre
  constraint coincident A35 L69.start
  constraint coincident L69.start L73.start
  constraint equal L69 L73
  constraint equal L71 L73
  constraint coincident L68.start L72.start
  measures "d281" distance of L1 L11
  measures "d282" distance of origin L11
  measures "d283" distance of L0.end P1
  measures "d284" distance of L0 L9.end
  measures "d285" distance of L0 L8
  measures "d286" distance of L0.start L1.end
  measures "d287" distance of L0 P0
  measures "d288" distance of L0 L6
  measures "d289" distance of L9.end L11
  measures "d290" distance of L8.end L11
  measures "d291" distance of L1 P0
  measures "d292" distance of L1 L3.end
  measures "d293" angle of L6 L7
  measures "d294" angle of L5 L6
  measures "d295" horizontal distance of origin L7.end
  measures "d296" horizontal distance of origin L4.end
  measures "d297" radius of A4
  measures "d298" radius of A5
  measures "d299" diameter of A6
  measures "d300" diameter of A7
  measures "d301" diameter of A8
  measures "d302" distance of L0 A7.centre
  measures "d303" distance of A7.centre A8.centre
  measures "d304" distance of L11 A8.centre
  measures "d306" distance of L20 L21
  measures "d307" radius of A9
  measures "d308" radius of A10
  measures "d309" distance of L0 L20
  measures "d310" distance of L20.start L20.end
  measures "d311" horizontal distance of origin L20.end
  measures "d312" radius of A13
  measures "d313" distance of L1 L12
  measures "d314" distance of L12 L25
  measures "d315" distance of L0 L14
  measures "d316" angle of L0 L15
  measures "d317" angle of L12 L13
  measures "d318" horizontal distance of origin L16.end
  measures "d319" horizontal distance of origin L13.end
  measures "d320" distance of origin L27
  measures "d321" distance of origin L26
  measures "d322" distance of origin L28
  measures "d323" distance of L1 A6.centre
  measures "d324" distance of L0 A6.centre
  measures "d369" diameter of A33
  measures "d370" diameter of A34
  measures "d371" diameter of A35
  measures "d374" diameter of A37
  measures "d376" diameter of A38
  measures "d377" diameter of A39
  measures "d379" diameter of A41
  measures "d380" diameter of A40
extrude "Extrude1''''''" add sketch "Profile (5)" along normal blind 2 separate body contours L1 L2 L3 L4 L5 L6 L7 L8 L9 L10 L11 A4 A5 L34 L39 L42 A20 L46 L50 L54 L57 L58 A29 L60 L63 L64 | L66 L67 L76 L77 L78 L88 | L68 L69 L70 L71 L72 L73 | L80 L81 L82 L83 L85 L86 | L89 L90 L91 L93 L95 L96 makes body 41 in component "Accessory Plate"
extrude "Extrude2''''" add sketch "Profile (3)" against normal blind 19 separate body contours A53 | A55 | A57 | A59 | A61 | A63 | A65 | A67 makes body 42 at (-151.4298, 19.451, 8.3333) makes body 43 at (151.4202, -24.499, 8.3333) makes body 44 at (151.4202, 18.101, 8.3333) makes body 45 at (-151.4298, -25.849, 8.3333) makes body 46 at (-104.8841, 47.8686, 8.3333) makes body 47 at (87.5159, -41.1564, 8.3333) makes body 48 at (90.1443, 38.3236, 8.3333) makes body 49 at (-104.8841, -47.2314, 8.3333) in component "Top Plate"
extrude "Extrude2'''''" add sketch "Profile (4)" against normal blind 10 separate body contours A4 | A5 | A6 A32 A47 | A7 A36 | L53 L54 L55 L56 L57 L58 | L59 L60 L61 L63 L65 L66 | L68 L70 L71 L72 L73 L74 | L76 L77 L78 L79 L80 L82 makes body 50 at (45.6746, 37.9275, 26.3333) makes body 51 at (45.6746, -37.0725, 26.3333) makes body 52 at (-66.6614, 38.7033, 26.3333) makes body 53 at (-66.6614, -36.2967, 26.3333) in component "Pixhawk Plate"
extrude "Extrude2''''''" add sketch "Profile (5)" against normal blind 15 separate body contours A0 | A1 A18 A36 | A2 A31 | A3 | L66 L67 L76 L77 L78 L88 | L68 L69 L70 L71 L72 L73 | L80 L81 L82 L83 L85 L86 | L89 L90 L91 L93 L95 L96 makes body 54 at (29.6438, 33.8755, 45) makes body 55 at (29.6438, -34.1245, 45) makes body 56 at (-41.0754, 33.5725, 40) makes body 57 at (-41.0754, -34.4275, 40) in component "Accessory Plate"